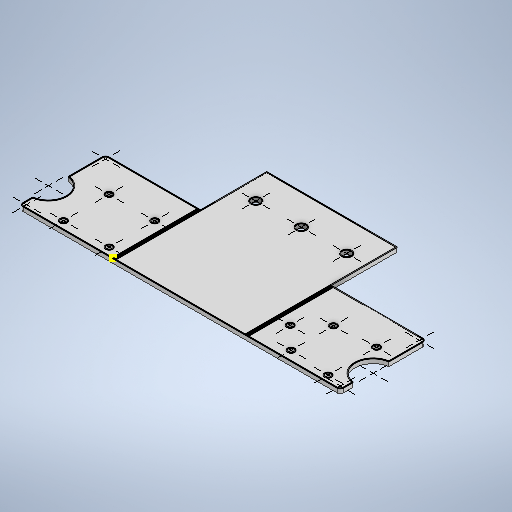
# Autodesk Inventor part: axis_23_top_frame
Saved by Autodesk Inventor 2025.2 (Build 292293000, 293)
## iProperties
Created: 2025-08-10
Part Number: axis_23_top_frame
Material: Generic
Document SubType Name: Modeling
Designer: LG
Density: 1 g/cm^3
Appearance: Default
Author: LG
Autodesk Inventor part; units mm, degrees
ref_plane "YZ Plane" through (0, 0, 0) normal (1, 0, 0) x (0, 1, 0)
ref_plane "XZ Plane" through (0, 0, 0) normal (0, 1, 0) x (-1, 0, 0)
ref_plane "XY Plane" through (0, 0, 0) normal (0, 0, 1) x (1, 0, 0)
sketch "Sketch1" plane through (0, 0, 0) normal (0, 1, 0) x (-1, 0, 0)
  line L0 (-44.2289, 0) -> (-44.2289, -28.14)
  line L1 (-0.4496, -28.14) -> (-0.4496, 0)
  circle A0 centre (-37.3393, -39.96) radius 1.55
  circle A1 centre (-22.3393, -39.96) radius 1.55
  circle A2 centre (-7.3393, -39.96) radius 1.55
  circle A3 centre (-48.5486, -10.07) radius 1.05
  circle A4 centre (-55.8486, -17.07) radius 1.05
  circle A5 centre (-55.8486, -3.07) radius 1.05
  circle A6 centre (-69.0686, -18.07) radius 1.05
  circle A7 centre (-69.0686, -2.07) radius 1.05
  circle A8 centre (18.79, -17.595) radius 1.05
  circle A9 centre (18.79, -2.545) radius 1.05
  circle A10 centre (3.69, -17.595) radius 1.05
  circle A11 centre (3.69, -2.545) radius 1.05
  arc A12 (30.49, -1) -> (29.49, 0) centre (29.49, -1) ccw
  line L2 (30.49, -1) -> (30.49, -4.1236)
  arc A13 (29.49, -28.14) -> (30.49, -27.14) centre (29.49, -27.14) ccw
  line L3 (29.49, -28.14) -> (-0.8993, -28.14)
  arc A14 (-75.1686, -27.14) -> (-74.1686, -28.14) centre (-74.1686, -27.14) ccw
  line L4 (-75.1686, -27.14) -> (-75.1686, -16.0164)
  line L5 (-43.7793, -28.14) -> (-74.1686, -28.14)
  line L6 (-43.7793, -50) -> (-43.7793, -28.14)
  line L7 (-0.8993, -50) -> (-43.7793, -50)
  line L8 (-0.8993, -28.14) -> (-0.8993, -50)
  line L9 (30.49, -16.0164) -> (30.49, -27.14)
  arc A15 (30.49, -4.1236) -> (30.49, -16.0164) centre (31.29, -10.07) ccw
  line L10 (-74.1686, 0) -> (29.49, 0)
  arc A16 (-74.1686, 0) -> (-75.1686, -1) centre (-74.1686, -1) ccw
  line L11 (-75.1686, -4.1236) -> (-75.1686, -1)
  arc A17 (-75.1686, -16.0164) -> (-75.1686, -4.1236) centre (-75.9686, -10.07) ccw
  line L12 (-44.6786, -28.14) -> (-44.6786, 0)
  line L13 (-43.7793, 0) -> (-43.7793, -28.14)
  line L14 (-0.8993, -28.14) -> (-0.8993, 0)
  line L15 (0, 0) -> (0, -28.14)
  constraints: 32 end point, 18 centre point, 14 equal radius, 13 tangent, 12 point on circle, 12 vertical, 10 point on line, 9 parallel, 4 horizontal, 3 perpendicular, 1 collinear, 63 other
extrude "Extrusion1" add sketch "Sketch1" against normal blind 1.5
body "Solid1"
